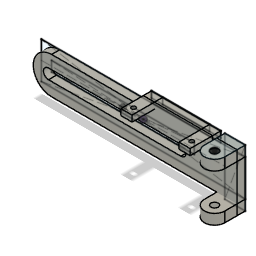
_PENARM.327dd406-160b-4e44-8dec-6c34584bab60 (Autodesk Fusion 360 design; units mm, degrees)
Autodesk Fusion 360 part; units mm, degrees
note: some values were not read from the file. Set by a fixed rule: which sketch regions a step uses.
sketch "Sketch1" plane through (0, 0, 0) normal (0, 0, 1) x (1, 0, 0)
  line L0 (50, -9) -> (-50, -9)
  line L1 (-50, -9) -> (-50, 9)
  line L2 (-50, 9) -> (50, 9)
  line L3 (50, 9) -> (50, -9)
  line L4 (50, -9) -> (-50, 9) construction
  line L5 (-50, -9) -> (50, 9) construction
  line L6 (40, 14) -> (50, 14)
  line L7 (50, 14) -> (50, -14)
  line L8 (50, -14) -> (40, -14)
  line L9 (40, -14) -> (40, 14)
  line L10 (4, 14) -> (38, 14)
  line L11 (38, 14) -> (38, 9)
  line L12 (38, 9) -> (4, 9)
  line L13 (4, 9) -> (4, 14)
  line L14 (38, 14) -> (4, 14)
  line L15 (4, 14) -> (4, 11)
  line L16 (4, 11) -> (38, 11)
  line L17 (38, 11) -> (38, 14)
  line L18 (9.5, 14) -> (32.5, 14)
  line L19 (32.5, 14) -> (32.5, 11)
  line L20 (32.5, 11) -> (9.5, 11)
  line L21 (9.5, 11) -> (9.5, 14)
  line L22 (50, 14) -> (40, -14) construction
  line L23 (-50, 0) -> (40, 0) construction
  line L24 (25, 2.5) -> (-45, 2.5)
  line L25 (-45, 2.5) -> (-45, -2.5)
  line L26 (-45, -2.5) -> (25, -2.5)
  line L27 (25, -2.5) -> (25, 2.5)
  line L28 (25, 2.5) -> (-45, -2.5) construction
  line L29 (-45, 2.5) -> (25, -2.5) construction
  point P0 (-10, 0)
  dimension "d1" = 100
  dimension "d2" = 18
  dimension "d3" = 28
  dimension "d4" = 10
  dimension "d5" = 5
  dimension "d6" = 34
  dimension "d7" = 3
  dimension "d8" = 5
  dimension "d9" = 5.5
  dimension "d10" = 5.5
  dimension "d12" = 2
  dimension "d13" = 70
  dimension "d14" = 5
  dimension "d15" = 5
  constraint horizontal L0
  constraint perpendicular L0 L1
  constraint parallel L0 L2
  constraint parallel L1 L3
  constraint coincident L4 origin
  constraint coincident L5 origin
  constraint horizontal L6
  constraint vertical L7
  constraint horizontal L8
  constraint vertical L9
  constraint horizontal L10
  constraint vertical L11
  constraint horizontal L12
  constraint vertical L13
  constraint coincident L2 L11.end
  constraint horizontal L14
  constraint vertical L15
  constraint horizontal L16
  constraint vertical L17
  constraint coincident L13 L15.end
  constraint horizontal L18
  constraint vertical L19
  constraint horizontal L20
  constraint vertical L21
  constraint coincident L16 L19.end
  constraint coincident L14 L18.start
  constraint midpoint L1 L23.start
  constraint coincident L9 L23.end
  constraint perpendicular L9 L23
  constraint collinear L3 L7
  constraint horizontal L24
  constraint perpendicular L24 L25
  constraint parallel L24 L26
  constraint parallel L25 L27
  constraint coincident L28 P0
  constraint coincident L29 P0
  constraint coincident L23 P0
  measures "d1" distance of L1.end L2.end
  measures "d2" distance of L0.end L1.end
  measures "d3" distance of L6.end L7.end
  measures "d4" distance of L6.start L6.end
  measures "d5" distance of L10.start L12.end
  measures "d6" distance of L10.start L10.end
  measures "d7" distance of L14 L16
  measures "d8" distance of L2 L6
  measures "d9" distance of L15 L21
  measures "d10" distance of L11 L19
  measures "d12" distance of L9 L11
  measures "d13" distance of L25.end L26.end
  measures "d14" distance of L24.end L25.end
  measures "d15" distance of L1 L25
extrude "Extrude1" add sketch "Sketch1" along normal blind 4 makes body 1
extrude "Extrude2" add sketch "Sketch1" along normal blind 15 separate body contours L0 L7 L8 L9 | L2 L6 L7 L9 | L10 L11 L14 L16 L17 L19 | L10 L13 L14 L15 L16 L21 makes body 2 at (46.6667, -14, 5) makes body 3 at (34.3333, 11, 5) makes body 4 at (43.3333, 9, 5) makes body 5 at (5.8333, 14, 5)
fillet "Fillet1" radius 5 4 edges at (40, -11.5, 15) (50, -11.5, 15) (40, 11.5, 15) (50, 11.5, 15) on bodies 2 4
fillet "Fillet2" radius 9 2 edges at (-50, 9, 2) (-50, -9, 2) on bodies 1
fillet "Fillet3" radius 2.5 4 edges at (-45, 2.5, 2) (-45, -2.5, 2) (25, 2.5, 2) (25, -2.5, 2) on bodies 1
sketch "Sketch2" plane through (0, 14, 0) normal (0, 1, 0) x (-1, 0, 0)
  arc A0 (-40, 10) -> (-50, 10) centre (-45, 10) ccw
  line L0 (-50, 10) -> (-50, 0)
  line L1 (-50, 0) -> (-40, 0)
  line L2 (-40, 0) -> (-40, 10)
  circle A1 centre (-45, 10) radius 1.75
  dimension "d26" = 3.5
  constraint concentric A0 A1
  measures "d26" diameter of A1
extrude "Extrude3" cut sketch "Sketch2" against normal through all contours A1 bodies 2 4
sketch "Sketch3" plane through (0, 14, 0) normal (0, 1, 0) x (-1, 0, 0)
  line L0 (-9.5, 0) -> (-4, 0)
  line L1 (-4, 0) -> (-4, 15)
  line L2 (-4, 15) -> (-9.5, 15)
  line L3 (-9.5, 15) -> (-9.5, 0)
  line L4 (-6.75, 15) -> (-6.75, 9)
  line L5 (-35.25, 17.6448) -> (-35.25, 12.3552)
  line L6 (-38, 15) -> (-32.5, 15)
  circle A0 centre (-35.25, 11.5) radius 1
  circle A1 centre (-6.75, 11.5) radius 1
  line L7 (-1, 11.5) -> (-39, 11.5) construction
  dimension "d28" = 3.5
  dimension "d29" = 2
  dimension "d30" = 2
  constraint midpoint L2 L4.start
  constraint perpendicular L2 L4
  constraint vertical L5
  constraint midpoint L5 L6
  constraint coincident L4 A1.centre
  constraint perpendicular L3 L7
  constraint coincident A1.centre L7
  constraint coincident A0.centre L7
  constraint coincident L5 A0.centre
  measures "d28" distance of L2 L7
  measures "d29" diameter of A1
  measures "d30" diameter of A0
extrude "Extrude4" cut sketch "Sketch3" against normal through all contours L4 A1 | L4 A1 | A0 bodies 3 5
equation "d30 = d29"
